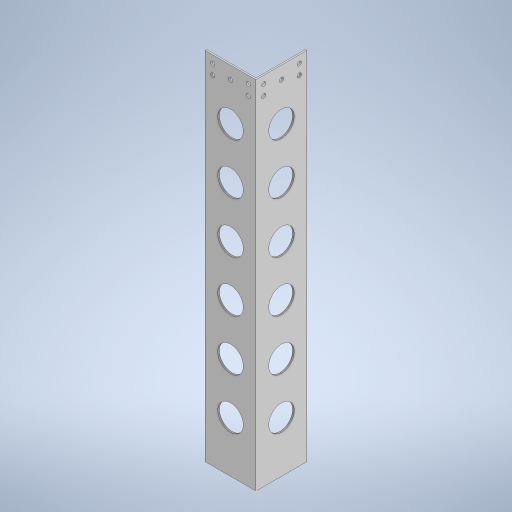
# Autodesk Inventor part: mesa completa
Saved by Autodesk Inventor 2024 (Build 280153000, 153)
## iProperties
Created: 2023-10-22
Part Number: mesa completa
Material: Genérico
Document SubType Name: Modeling
Designer: jhonc
Density: 1 g/cm^3
Appearance: Valor por defecto
Author: jhonc
Autodesk Inventor part; units mm, degrees
ref_plane "YZ Plane" through (0, 0, 0) normal (1, 0, 0) x (0, 1, 0)
ref_plane "XZ Plane" through (0, 0, 0) normal (0, 1, 0) x (-1, 0, 0)
ref_plane "XY Plane" through (0, 0, 0) normal (0, 0, 1) x (1, 0, 0)
sketch "Boceto6" plane through (0, 0, 0) normal (0, 1, 0) x (-1, 0, 0)
  line L0 (0, 0) -> (100, 0)
  line L1 (100, 0) -> (100, -100)
  line L2 (100, -100) -> (0, -100)
  line L3 (0, -100) -> (0, 0)
  line L4 (97, -97) -> (97, -3)
  line L5 (97, -3) -> (3, -3)
  line L6 (3, -3) -> (3, -97)
  line L7 (3, -97) -> (97, -97)
  line L8 (97, -3) -> (100, -3)
  line L9 (3, -97) -> (3, -106.6251)
  point P0 (3, -100)
  dimension "d46" = 100
  dimension "d47" = 100
  dimension "d48" = 3
  constraints: 20 end point, 4 parallel, 4 perpendicular, 1 horizontal, 1 point on line, 3 other
  measures "d46" distance of L0.start L0.end
  measures "d47" distance of L2.end L0.start
  measures "d48" distance between parallel lines of L1 L4
extrude "Extrusión6" add sketch "Boceto6" along normal blind 700 contours L0 L1 L8 L5 L6 L9 L2 L3
sketch "Boceto7" plane through (0, 0, 0) normal (1, 0, 0) x (0, 0, -1)
  line L0 (100, 0) -> (100, 700) projected
  line L1 (0, 700) -> (100, 700)
  line L2 (100, 700) -> (100, 650)
  line L3 (100, 650) -> (0, 650)
  line L4 (0, 650) -> (0, 700)
  circle A0 centre (50, 600) radius 25
  circle A1 centre (50, 500) radius 25
  circle A2 centre (50, 400) radius 25
  circle A3 centre (50, 300) radius 25
  circle A4 centre (50, 200) radius 25
  circle A5 centre (50, 100) radius 25
  circle A6 centre (15, 685) radius 4
  circle A7 centre (85, 685) radius 4
  circle A8 centre (15, 665) radius 4
  circle A9 centre (85, 665) radius 4
  circle A10 centre (50, 675) radius 4
  line L5 (0, 700) -> (100, 700) projected
  point P0 (0, 0)
  point P1 (50, 650)
  point P2 (50, 700)
  dimension "d51" = 50
  dimension "d52" = 50
  dimension "d53" = 50
  dimension "d54" = 50
  dimension "d57" = 100
  dimension "d62" = 8
  dimension "d64" = 15
  dimension "d65" = 15
  dimension "d66" = 8
  dimension "d67" = 8
  dimension "d68" = 8
  dimension "d69" = 15
  dimension "d70" = 15
  dimension "d71" = 15
  dimension "d72" = 15
  dimension "d73" = 15
  dimension "d74" = 15
  dimension "d75" = 8
  dimension "d76" = 25
  dimension "d77" = 50
  dimension "d110" = 0
  constraints: 11 centre point, 8 end point, 2 midpoint, 2 parallel, 1 horizontal, 1 perpendicular, 1 point on line, 1 vertical, 10 other
  measures "d51" distance between parallel lines of L3 L1
  measures "d52" diameter of A0
  measures "d53" distance of A0.centre point (50, 650)
  measures "d54" distance from line of L0 A0.centre
  measures "d57" distance of A0.centre A1.centre
  measures "d62" diameter of A6
  measures "d64" distance from line of L1 A6.centre
  measures "d65" distance from line of L4 A6.centre
  measures "d66" diameter of A7
  measures "d67" diameter of A8
  measures "d68" diameter of A9
  measures "d69" distance from line of L1 A7.centre
  measures "d70" distance from line of L2 A7.centre
  measures "d71" distance from line of L0 A9.centre
  measures "d72" distance from line of L3 A9.centre
  measures "d73" distance from line of L4 A8.centre
  measures "d74" distance from line of L3 A8.centre
  measures "d75" diameter of A10
  measures "d76" distance from line of L1 A10.centre
  measures "d77" distance from line of L4 A10.centre
  measures "d110" distance from line of point (50, 700) L1
extrude "Extrusión7" cut sketch "Boceto7" against normal blind 700 contours A0 | A1 | A2 | A3 | A4 | A5 | A6 | A7 | A8 | A9 | A10
sketch "Boceto8" plane through (-100, 0, 0) normal (0, 0, 1) x (1, 0, 0)
  line L0 (100, -78.2713) -> (100, 621.7287)
  line L1 (0, 700) -> (100, 700)
  line L2 (100, 700) -> (100, 650)
  line L3 (100, 650) -> (0, 650)
  line L4 (0, 650) -> (0, 700)
  circle A0 centre (50, 600) radius 25
  circle A1 centre (50, 500) radius 25
  circle A2 centre (50, 400) radius 25
  circle A3 centre (50, 300) radius 25
  circle A4 centre (50, 200) radius 25
  circle A5 centre (50, 100) radius 25
  circle A6 centre (15, 685) radius 4
  circle A7 centre (85, 685) radius 4
  circle A8 centre (15, 665) radius 4
  circle A9 centre (85, 665) radius 4
  circle A10 centre (50, 675) radius 4
  line L5 (0, 0) -> (0, 700) projected
  line L6 (100, 0) -> (100, 700) projected
  line L7 (0, 700) -> (100, 700) projected
  point P0 (4.2464, -128.2713)
  point P1 (50, 650)
  dimension "d84" = 50
  dimension "d85" = 50
  dimension "d86" = 50
  dimension "d87" = 50
  dimension "d88" = 100
  dimension "d89" = 8
  dimension "d90" = 15
  dimension "d91" = 15
  dimension "d92" = 8
  dimension "d93" = 8
  dimension "d94" = 8
  dimension "d95" = 15
  dimension "d96" = 15
  dimension "d97" = 15
  dimension "d98" = 15
  dimension "d99" = 15
  dimension "d100" = 15
  dimension "d101" = 8
  dimension "d102" = 25
  dimension "d103" = 50
  dimension "d105" = 0
  dimension "d106" = 0
  dimension "d107" = 0
  constraints: 11 centre point, 10 end point, 2 parallel, 1 horizontal, 1 midpoint, 1 perpendicular, 1 point on line, 1 vertical, 10 other
  measures "d84" distance between parallel lines of L3 L1
  measures "d85" diameter of A0
  measures "d86" distance of A0.centre point (50, 650)
  measures "d87" distance from line of L0 A0.centre
  measures "d88" distance of A0.centre A1.centre
  measures "d89" diameter of A6
  measures "d90" distance from line of L1 A6.centre
  measures "d91" distance from line of L4 A6.centre
  measures "d92" diameter of A7
  measures "d93" diameter of A8
  measures "d94" diameter of A9
  measures "d95" distance from line of L1 A7.centre
  measures "d96" distance from line of L2 A7.centre
  measures "d97" distance from line of L0 A9.centre
  measures "d98" distance from line of L3 A9.centre
  measures "d99" distance from line of L4 A8.centre
  measures "d100" distance from line of L3 A8.centre
  measures "d101" diameter of A10
  measures "d102" distance from line of L1 A10.centre
  measures "d103" distance from line of L4 A10.centre
  measures "d105" distance between parallel lines of L5 L4
  measures "d106" distance between parallel lines of L6 L2
  measures "d107" distance between parallel lines of L7 L1
extrude "Extrusión8" cut sketch "Boceto8" against normal blind 700 contours A0 | A1 | A2 | A3 | A4 | A5 | A6 | A7 | A8 | A9 | A10
sketch "Boceto9" plane through (-100, 0, 0) normal (0, 0, 1) x (1, 0, 0)
  point P0 (100, 0)
